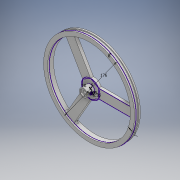
# Autodesk Inventor part: bigWheel
Saved by Autodesk Inventor 2018 (Build 220112000, 112)
## iProperties
Created: 2017-10-25
Part Number: bigWheel
Material: Generic
Document SubType Name: Modeling
Designer: Payal Jindal
Density: 1 g/cm^3
Appearance: Default
Author: Payal Jindal
Autodesk Inventor part; units mm, degrees
ref_plane "XZ Plane" through (0, 0, 0) normal (0, 1, 0) x (-1, 0, 0)
ref_plane "XY Plane" through (0, 0, 0) normal (0, 0, 1) x (1, 0, 0)
sketch "Sketch1" plane through (0, 0, 0) normal (0, 1, 0) x (-1, 0, 0)
  circle A0 centre (0, 0) radius 90
  circle A1 centre (0, 0) radius 88
  circle A2 centre (0, 0) radius 82
  circle A3 centre (0, 0) radius 3.175
  circle A4 centre (0, 0) radius 8.175
  circle A5 centre (0, 0) radius 18.175
  line L0 (-15.740012, -9.0875) -> (-15.740012, 9.0875)
  line L1 (-15.740012, 9.0875) -> (0, 18.175)
  line L2 (0, 18.175) -> (15.740012, 9.0875)
  line L3 (15.740012, 9.0875) -> (15.740012, -9.0875)
  line L4 (15.740012, -9.0875) -> (0, -18.175)
  line L5 (0, -18.175) -> (-15.740012, -9.0875)
  line L6 (-15.740012, 9.0875) -> (-81.494892, 9.0875)
  line L7 (-15.740012, -9.0875) -> (-81.494892, -9.0875)
  arc A6 (-81.494892, 9.0875) -> (-81.494892, -9.0875) centre (0, 0) ccw
  arc A7 (-15.740012, 9.0875) -> (-15.740012, -9.0875) centre (0, 0) ccw
  dimension "d3" = 2
  dimension "d6" = 8
  dimension "d11" = 6.35
  dimension "d14" = 5
  dimension "d35" = 10
  dimension "d78" = 176
  constraints: 16 end point, 7 centre point, 7 coincident, 6 point on circle, 1 concentric, 1 horizontal, 1 parallel, 1 vertical, 17 other
  measures "d3" radial gap between concentric circles of A0 A1
  measures "d6" radial gap between concentric circles of A2 A0
  measures "d11" diameter of A3
  measures "d14" radial gap between concentric circles of A4 A3
  measures "d78" diameter of A1
extrude "Extrusion2" add sketch "Sketch1" along normal blind 5.7625 contours A1 | A2 L7 A5 L6 | L6 A5 L7 A2 | L0 A5 | L1 L2 L3 L4 L5 L0 | A5 L1 | L5 A5 | A5 L2 | L4 A5 | A5 L3 | A3 | A4
extrude "Extrusion3" add sketch "Sketch1" against normal blind 3 contours A0 | A1
sketch "Sketch3" plane through (0, 5.7625, 0) normal (0, 1, 0) x (1, 0, 0)
  circle A0 centre (0, 0) radius 82 projected
  circle A1 centre (0, 0) radius 90 projected
extrude "Extrusion4" add sketch "Sketch3" along normal blind 3
extrude "Extrusion5" cut sketch "Sketch1" along normal blind 35.75 contours A3
extrude "Extrusion6" add sketch "Sketch1" against normal blind 14 contours A4
ref_plane "Work Plane1" through (8.175, 0, 0) normal (1, 0, 0) x (0, 1, 0)
sketch "Sketch5" plane through (8.175, 0, 0) normal (1, 0, 0) x (0, 1, 0)
  line L0 (-14, -3.175) -> (-14, 3.175) construction
  line L1 (-14, 0) -> (0, 0) construction
  circle A0 centre (-7, 0) radius 2.6543
  circle A1 centre (-7, 0) radius 2.5273
  circle A2 centre (-7, 0) radius 1.8
  dimension "d49" = 5.3086
  dimension "d50" = 5.0546
  dimension "d80" = 3.6
  constraints: 3 centre point, 2 coincident, 2 end point, 2 midpoint, 1 horizontal
  measures "d49" diameter of A0
  measures "d50" diameter of A1
  measures "d80" diameter of A2
extrude "Extrusion9" cut sketch "Sketch5" against normal blind 3.81 contours A1 | A2
loft "Loft1" cut profiles "Sketch5" section 2 edges at (4.365, -9.5273, 0) contours A0 | A1 | A2
sketch "Sketch6" plane through (0, -14, 0) normal (0, -1, 0) x (1, 0, 0)
  line L0 (-6.05625, 3.496578) -> (0, 6.993155)
  line L1 (0, 6.993155) -> (6.05625, 3.496578)
  line L2 (6.05625, 3.496578) -> (6.05625, -3.496578)
  line L3 (6.05625, -3.496578) -> (0, -6.993155)
  line L4 (0, -6.993155) -> (-6.05625, -3.496578)
  line L5 (-6.05625, -3.496578) -> (-6.05625, 3.496578)
  point P0 (0, 0)
  point P1 (0, 0)
  dimension "d57" = 12.1125
  constraints: 12 end point, 1 coincident, 1 vertical, 13 other
  measures "d57" distance between parallel lines of L5 L2
extrude "Extrusion10" cut sketch "Sketch6" against normal blind 3
sketch "Sketch7" plane through (0, 5.7625, 0) normal (0, 1, 0) x (1, 0, 0)
  circle A0 centre (0, 0) radius 13
  dimension "d67" = 26
  constraints: 1 centre point, 1 coincident
  measures "d67" diameter of A0
extrude "Extrusion12" cut sketch "Sketch7" against normal blind 2
extrude "Extrusion13" cut sketch "Sketch1" along normal up to surface (5.7625 mm away) contours A2 L7 A5 L6 | L6 A5 L7 A2
extrude "Extrusion14" add sketch "Sketch1" along normal up to surface (5.7625 mm away) from surface at 0 contours L6 A5 L7 A2 picked at (-60.654362, 0.633268)
pattern_circular "Circular Pattern2" count 3 over 360 about axis through (0, 0, 0) along (0, 1, 0) of "Extrusion14"
fillet "Fillet1" radius 3 6 edges at (-48.6175, 2.8812, -66.0329) (-48.6175, 2.8813, 66.0329) (-32.8774, 2.8813, 75.1204) (-32.8774, 2.8812, -75.1204) (81.4949, 2.8813, -9.0875) (81.4949, 2.8813, 9.0875)
extrude "Extrusion15" cut sketch "Sketch5" against normal up to surface contours A2
body "Solid2"
